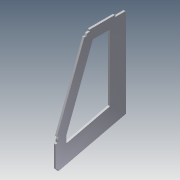
# Autodesk Inventor part: TopSidePanel
Saved by Autodesk Inventor 2014 (Build 180170000, 170)
## iProperties
Created: 2014-08-11
Part Number: TopSidePanel
Material: Generic
Document SubType Name: Modeling
Designer: Peele
Density: 1 g/cm^3
Appearance: White
Author: Peele
Autodesk Inventor part; units mm, degrees
ref_plane "YZ Plane" through (0, 0, 0) normal (1, 0, 0) x (0, 1, 0)
ref_plane "XZ Plane" through (0, 0, 0) normal (0, 1, 0) x (-1, 0, 0)
ref_plane "XY Plane" through (0, 0, 0) normal (0, 0, 1) x (1, 0, 0)
sketch "Sketch1" plane through (0, 0, 0) normal (1, 0, 0) x (0, 1, 0)
  line L0 (0, 325) -> (0, 0)
  line L1 (0, 0) -> (-211, 0)
  line L2 (-211, 0) -> (-211, 85)
  line L3 (-2.4145, 325) -> (0, 325)
  line L4 (0, 325) -> (-120, 325)
  line L5 (-120, 325) -> (-211, 85)
  dimension "d0" = 325
  dimension "d1" = 211
  dimension "d2" = 85
  dimension "d3" = 120
  dimension "d33" = 240
  dimension "d34" = 91
  constraints: 12 end point, 2 parallel, 1 collinear, 1 perpendicular, 1 vertical
  measures "d0" distance of L0.start L0.end
  measures "d1" distance of L0.end L1.end
  measures "d2" distance of L1.end L2.end
  measures "d3" distance of L0.start L4.end
  measures "d33" vertical distance of L2.end L4.end
  measures "d34" horizontal distance of L4.end L2.end
extrude "Extrusion1" add sketch "Sketch1" along normal blind 6
sketch "Sketch2" plane through (6, 0, 0) normal (1, 0, 0) x (0, 0, -1)
  line L0 (-325, 0) -> (-325, -120) projected
  line L1 (-325, -33.1) -> (-331, -33.1)
  line L2 (-331, -33.1) -> (-331, -111.9)
  line L3 (-331, -111.9) -> (-325, -111.9)
  line L4 (-325, -111.9) -> (-325, -33.1)
  line L5 (-85, -211) -> (0, -211) projected
  line L6 (0, -211) -> (0, 0) projected
  line L7 (-76.9, -211) -> (-8.1, -211)
  line L8 (-8.1, -211) -> (-8.1, -217)
  line L9 (-8.1, -217) -> (-76.9, -217)
  line L10 (-76.9, -217) -> (-76.9, -211)
  line L11 (-325, -120) -> (-331, -111.9) construction
  line L12 (0, 0) -> (-325, 0) projected
  line L13 (-325, -25) -> (-331, -33.1) construction
  dimension "d6" = 6
  dimension "d12" = 6
  dimension "d13" = 8.1
  dimension "d38" = 25
  dimension "d47" = 8.1
  dimension "d48" = 8.1
  constraints: 20 end point, 4 parallel, 3 point on line, 2 horizontal, 2 perpendicular, 1 equal length
  measures "d6" distance of L1.start L1.end
  measures "d12" distance of L7.end L8.end
  measures "d13" distance between parallel lines of L8 L6
  measures "d38" distance from line of L13.start L12
  measures "d47" distance from line of L5.start L10
  measures "d48" distance from line of L0.end L3
extrude "Extrusion2" add sketch "Sketch2" against normal blind 6
sketch "Sketch3" plane through (6, 0, 0) normal (1, 0, 0) x (0, 0, -1)
  line L0 (-317.4262, -122.8717) -> (-92.5738, -208.1283)
  line L1 (-92.5738, -208.1283) -> (-94.7011, -213.7385)
  line L2 (-94.7011, -213.7385) -> (-319.5534, -128.482)
  line L3 (-319.5534, -128.482) -> (-317.4262, -122.8717)
  line L4 (-325, -120) -> (-85, -211) projected
  dimension "d17" = 8.1
  dimension "d35" = 6
  dimension "d36" = 8.1
  constraints: 8 end point, 2 parallel, 1 collinear, 1 perpendicular
  measures "d17" distance from line of L4.start L3
  measures "d35" distance between parallel lines of L2 L0
  measures "d36" distance from line of L4.end L1
extrude "Extrusion3" add sketch "Sketch3" against normal blind 6
sketch "Sketch6" plane through (6, 0, 0) normal (1, 0, 0) x (0, 0, -1)
  line L0 (0, 0) -> (-325, 0) projected
  line L1 (0, -211) -> (0, 0) projected
  line L2 (0, -211) -> (-50, 0)
  line L3 (-50, 0) -> (0, 0)
  line L4 (0, -211) -> (0, 0)
  dimension "d39" = 50
  constraints: 6 end point, 2 perpendicular, 1 point on line
  measures "d39" distance of L2.end L0.start
extrude "Extrusion6" cut sketch "Sketch6" against normal through all
fillet "Fillet2" radius 3 4 edges at (3, 0, 325) (3, -120, 325) (3, -211, 85) (3, -211, 0)
fillet "Fillet3" radius 2 6 edges at (3, -217, 8.1) (3, -217, 76.9) (3, -213.7385, 94.7011) (3, -128.482, 319.5534) (3, -111.9, 331) (3, -33.1, 331)
sketch "Sketch4" plane through (6, 0, 0) normal (1, 0, 0) x (0, 0, -1)
  line L0 (-323.0636, -120.7342) -> (-85.514, -210.8051) projected
  line L1 (-323.0636, -120.7342) -> (-85.514, -210.8051) projected
  line L2 (-50, 0) -> (-322, 0) projected
  line L3 (-325, -3) -> (-325, -33.1) projected
  line L4 (-325, -33.1) -> (-329, -33.1) projected
  line L5 (-300, -50) -> (-300, -102.7424)
  line L6 (-300, -102.7424) -> (-84.4503, -184.4716)
  line L7 (-84.4503, -184.4716) -> (-84.4503, -50)
  line L8 (-84.4503, -50) -> (-300, -50)
  arc A0 (-85.514, -210.8051) -> (-84.4503, -211) centre (-84.4503, -208) ccw projected
  point P0 (-191.5213, -165.6514)
  point P1 (-106.0854, -201.6057)
  point P2 (-3, 0)
  point P3 (0, 0)
  dimension "d24" = 50
  dimension "d26" = 25
  dimension "d27" = 25
  constraints: 8 end point, 1 parallel, 1 perpendicular, 1 vertical alignment, 3 other
  measures "d24" distance between parallel lines of L2 L8
  measures "d27" distance between parallel lines of L3 L5
extrude "Extrusion4" cut sketch "Sketch4" against normal through all
sketch "Sketch7" plane through (6, 0, 0) normal (1, 0, 0) x (0, 0, -1)
  line L0 (-0.8748, -207.3083) -> (-50, 0) projected
  line L1 (-325, -33.1) -> (-329, -33.1) projected
  line L2 (-84.4503, -50) -> (-52.585, -184.4716)
  line L3 (-52.585, -184.4716) -> (-84.4503, -184.4716)
  line L4 (-84.4503, -50) -> (-84.4503, -184.4716)
  point P0 (0, 0)
  constraints: 6 end point, 2 parallel, 1 perpendicular
extrude "Extrusion7" cut sketch "Sketch7" against normal through all
sketch "Sketch8" plane through (6, 0, 0) normal (1, 0, 0) x (0, 0, -1)
  line L0 (-84.4503, -50) -> (-52.585, -184.4716) projected
  line L1 (-300, -50) -> (-84.4503, -50) projected
  line L2 (-52.585, -184.4716) -> (-84.4503, -50)
  line L3 (-84.4503, -50) -> (-94.4503, -50)
  line L4 (-94.4503, -50) -> (-62.585, -184.4716)
  line L5 (-52.585, -184.4716) -> (-62.585, -184.4716)
  line L6 (-52.585, -184.4716) -> (-84.4503, -184.4716) projected
  point P0 (0, 0)
  dimension "d44" = 10
  constraints: 8 end point, 2 equal length, 1 collinear, 1 point on line
  measures "d44" distance of L0.end L4.end
extrude "Extrusion8" add sketch "Sketch8" against normal blind 6
fillet "Fillet4" radius 2 5 edges at (3, -184.4716, 62.585) (3, -184.4716, 84.4503) (3, -50, 94.4503) (3, -102.7424, 300) (3, -50, 300)
equation "\"d26\" = d27"
body "Solid1"
